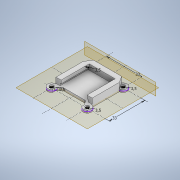
# Autodesk Inventor part: Electro_lora
Saved by Autodesk Inventor 2020 (Build 240168000, 168)
## iProperties
Created: 2020-09-03
Part Number: Electro_lora
Material: Generisch
Document SubType Name: Modeling
Designer: sp
Density: 1 g/cm^3
Appearance: Vorgabe
Author: sp
## iProperties of the stored document _3D-Druck.ipt
Created: 2022-05-23
Part Number: _3D-Druck
Material: Generisch
Document SubType Name: Modeling
Designer: sp
Density: 1 g/cm^3
Appearance: Vorgabe
Author: sp
Autodesk Inventor part; units mm, degrees
ref_plane "YZ Plane" through (0, 0, 0) normal (1, 0, 0) x (0, 1, 0)
sketch "Skizze1" plane through (0, 0, 0) normal (0, 1, 0) x (-1, 0, 0)
  circle A0 centre (0, 0) radius 30
  circle A1 centre (0, 0) radius 27
  dimension "d0" = 60
  dimension "d1" = 54
  constraints: 2 centre point, 2 coincident
  measures "d0" diameter of A0
  measures "d1" diameter of A1
extrude "Extrusion1" add sketch "Skizze1" along normal mid plane 10
sketch "Skizze5" plane through (0, 0, 0) normal (0, 1, 0) x (-1, 0, 0)
  line L0 (12.75, -14.75) -> (-12.75, -14.75)
  line L1 (-12.75, -14.75) -> (-12.75, 14.75)
  line L2 (-12.75, 14.75) -> (12.75, 14.75)
  line L3 (12.75, 14.75) -> (12.75, -14.75)
  line L4 (49.4097, 0) -> (-52.5504, 0) construction
  line L5 (0, -53.7913) -> (0, 68.1535) construction
  line L6 (-16.75, -18.75) -> (16.75, -18.75)
  line L7 (16.75, -18.75) -> (16.75, 18.75)
  line L8 (16.75, 18.75) -> (-16.75, 18.75)
  line L9 (-16.75, 18.75) -> (-16.75, -18.75)
  point P0 (0, 0)
  dimension "d33" = 29.5
  dimension "d34" = 25.5
  dimension "d35" = 4
  constraints: 20 end point, 4 parallel, 2 horizontal, 2 perpendicular, 2 point on line, 1 vertical, 5 other
  measures "d33" distance of L0.end L1.end
  measures "d34" distance of L0.start L0.end
  measures "d35" distance between parallel lines of L0 L6
extrude "Extrusion5" add sketch "Skizze5" along normal mid plane 2.5 contours L0 L1 L2 L3 | L9 L8 L7 L6
ref_plane "Arbeitsebene1" through (0, 0, 0) normal (0, 1, 0) x (-1, 0, 0)
chamfer "Fase1" distance 1 angle 45 2 edges at (30, 5, 0) (30, -5, 0)
sketch "Skizze2" plane through (0, 0, 0) normal (0, 1, 0) x (-1, 0, 0)
  line L0 (0, 42.2301) -> (0, -36.7007) construction
  line L1 (32.6355, 0) -> (-32.6355, 0) construction
  line L2 (16.5, 34.419) -> (16.5, -40.3324) construction
  line L3 (-16.5, 35.4304) -> (-16.5, -34.8157) construction
  line L4 (23.5881, 16.5) -> (-32.0387, 16.5) construction
  line L5 (23.5881, -16.5) -> (-39.8541, -16.5) construction
  circle A0 centre (16.5, -16.5) radius 1.75
  circle A1 centre (16.5, 16.5) radius 1.75
  circle A2 centre (-16.5, 16.5) radius 1.75
  circle A3 centre (-16.5, -16.5) radius 1.75
  circle A4 centre (-16.5, 16.5) radius 3.6749
  circle A5 centre (-16.5, -16.5) radius 3.7161
  circle A6 centre (16.5, -16.5) radius 3.7
  circle A7 centre (16.5, 16.5) radius 3.6747
  point P0 (0, 0)
  dimension "d8" = 33
  dimension "d9" = 33
  dimension "d10" = 3.5
  dimension "d11" = 3.5
  dimension "d12" = 3.5
  dimension "d13" = 3.5
  constraints: 12 end point, 9 point on line, 8 centre point, 4 coincident, 3 horizontal, 3 vertical, 1 midpoint, 2 other
  measures "d8" distance between parallel lines of L3 L2
  measures "d9" distance between parallel lines of L4 L5
  measures "d10" diameter of A0
  measures "d11" diameter of A1
  measures "d12" diameter of A2
  measures "d13" diameter of A3
extrude "Extrusion2" add sketch "Skizze2" along normal mid plane 2.5
ref_plane "Arbeitsebene2" through (0, 0, -30.5) normal (0, 0, 1) x (1, 0, 0)
extrude "Extrusion6" cut sketch "Skizze2" against normal mid plane 3 contours A0 | A1 | A2 | A3
sketch "Skizze12" plane through (0, 5, 0) normal (0, 1, 0) x (1, 0, 0)
  circle A0 centre (0, 0) radius 27
  circle A1 centre (0, 0) radius 31.5802
  constraints: 2 centre point, 2 coincident
extrude "Extrusion13" cut sketch "Skizze12" against normal blind 10
sketch "Skizze13" plane through (0, 1.25, 0) normal (0, 1, 0) x (1, 0, 0)
  line L0 (-13.5947, -18.75) -> (13.5944, -18.75) projected
  line L1 (-13.5947, -18.75) -> (13.5944, -18.75)
  line L2 (13.5944, -18.75) -> (13.5944, -14.75)
  line L3 (13.5944, -14.75) -> (-13.5947, -14.75)
  line L4 (-13.5947, -14.75) -> (-13.5947, -18.75)
  point P0 (0, 0)
  dimension "d58" = 4
  constraints: 8 end point, 2 parallel, 1 horizontal, 1 perpendicular
  measures "d58" distance of L2.end L1.end
extrude "Extrusion14" cut sketch "Skizze13" against normal blind 3
sketch "Skizze14" plane through (0, 1.25, 0) normal (0, 1, 0) x (1, 0, 0)
  line L0 (-13, -12.25) -> (13, -12.25)
  line L1 (13, -12.25) -> (13, 13.75)
  line L2 (13, 13.75) -> (-13, 13.75)
  line L3 (-13, 13.75) -> (-13, -12.25)
  line L4 (0, -43.7267) -> (0, 49.5069) construction
  line L5 (-24.7381, 0) -> (29.5694, 0) construction
  line L6 (13.5425, 18.75) -> (-13.5627, 18.75) construction
  line L7 (-13, -12.25) -> (-16.75, -12.25)
  line L8 (-16.75, 12.8084) -> (-16.75, -12.8338) projected
  line L9 (-16.75, -12.25) -> (-16.75, 12.815)
  line L10 (-16.75, 12.815) -> (-13.0013, 18.75)
  line L11 (13, -12.25) -> (16.75, -12.25)
  line L12 (16.75, -12.8336) -> (16.75, 12.7924) projected
  arc A0 (16.75, 12.7924) -> (19.551, 18.6215) centre (16.5, 16.5) ccw projected
  line L13 (16.75, -12.25) -> (16.75, 12.7924)
  line L14 (16.75, 12.7924) -> (13.0013, 18.75)
  line L15 (13.0013, 18.75) -> (-13.0013, 18.75)
  point P0 (0, 0)
  dimension "d62" = 26
  dimension "d63" = 26
  dimension "d64" = 5
  constraints: 26 end point, 7 point on line, 3 horizontal, 3 vertical, 2 parallel, 1 perpendicular, 1 other
  measures "d62" distance of L0.end L1.end
  measures "d63" distance of L1.end L2.end
  measures "d64" distance between parallel lines of L6 L2
extrude "Extrusion15" add sketch "Skizze14" along normal blind 5 contours L7 L8 L9 L10 L15 L14 L12 L11 L1 L2 L3
sketch "Skizze15" plane through (0, 6.25, 0) normal (0, 1, 0) x (1, 0, 0)
  line L0 (-13, 13.75) -> (-13, -12.25) projected
  line L1 (13, 13.75) -> (-13, 13.75) projected
  line L2 (-13, -12.25) -> (-12, -12.25)
  line L3 (-12, -12.25) -> (-12, 13.75)
  line L4 (-12, 13.75) -> (-13, 13.75)
  line L5 (-13, 13.75) -> (-13, -12.25)
  line L6 (13, -12.25) -> (16.75, -12.25) projected
  line L7 (13, -12.25) -> (12, -12.25)
  line L8 (12, -12.25) -> (12, 13.75)
  line L9 (12, 13.75) -> (13, 13.75)
  line L10 (13, 13.75) -> (13, -12.25)
  point P0 (0, 0)
  dimension "d67" = 1
  dimension "d68" = 1
  constraints: 16 end point, 4 parallel, 2 horizontal, 2 perpendicular, 2 point on line
  measures "d67" distance of L4.end L3.end
  measures "d68" distance of L8.end L9.end
extrude "Extrusion16" add sketch "Skizze15" against normal blind 3
sketch "Skizze16" plane through (0, 1.25, 0) normal (0, 1, 0) x (1, 0, 0)
  line L0 (12, -12.25) -> (12, 13.75) projected
  line L1 (12, -12.25) -> (-12.0731, -12.25)
  line L2 (-12.0731, -12.25) -> (-12.0731, -16.1057)
  line L3 (-12.0731, -16.1057) -> (12, -16.1057)
  line L4 (12, -16.1057) -> (12, -12.25)
  point P0 (0, 0)
  constraints: 8 end point, 2 parallel, 1 horizontal, 1 perpendicular
extrude "Extrusion17" cut sketch "Skizze16" against normal blind 10
fillet "Rundung5" radius 2 6 edges at (-13.5947, 0, 14.75) (-12.0731, 0, 14.75) (-12.0731, 0, 12.25) (12, 0, 12.25) (12, 0, 14.75) (13.5944, 0, 14.75)
